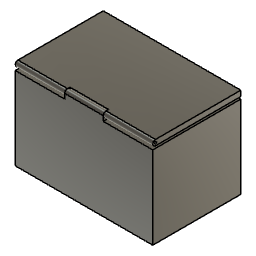
Speaker Holder Prototype v7 (Autodesk Fusion 360 design; units mm, degrees)
Autodesk Fusion 360 part; units mm, degrees
note: some values were not read from the file. Set by a fixed rule: which sketch regions a step uses.
sketch "Sketch1" plane through (0, 0, 0) normal (0, 0, 1) x (1, 0, 0)
  line L0 (-100, 50) -> (400, 50)
  line L1 (400, 50) -> (400, -150)
  line L2 (400, -150) -> (-100, -150)
  line L3 (-100, -150) -> (-100, 50)
  dimension "d1" = 500
  dimension "d2" = 200
  constraint horizontal L0
  constraint vertical L1
  constraint horizontal L2
  constraint vertical L3
  measures "d1" distance of L0.start L0.end
  measures "d2" distance of L0.start L2.end
extrude "Extrude1" add sketch "Sketch1" along normal blind 100 makes body 1
sketch "Sketch2" plane through (0, 0, 100) normal (0, 0, 1) x (-1, 0, 0)
  line L0 (100, 150) -> (-400, 150)
  line L1 (-400, 150) -> (-400, -50)
  line L2 (-400, -50) -> (100, -50)
  line L3 (100, -50) -> (100, 150)
  line L4 (90, -40) -> (-390, -40)
  line L5 (-390, -40) -> (-390, 140)
  line L6 (-390, 140) -> (90, 140)
  line L7 (90, 140) -> (90, -40)
  constraint horizontal L4
  constraint vertical L5
  constraint horizontal L6
  constraint vertical L7
extrude "Extrude2" cut sketch "Sketch2" against normal blind 90 contours L4 L5 L6 L7 bodies 1
sketch "Sketch3" plane through (0, 0, 100) normal (0, 0, 1) x (-1, 0, 0)
  line L0 (-390, -40) -> (-390, 140)
  line L1 (-390, 140) -> (90, 140)
  line L2 (90, 140) -> (90, -40)
  line L3 (90, -40) -> (-390, -40)
  line L4 (100, 150) -> (-400, 150)
  line L5 (-400, 150) -> (-400, -50)
  line L6 (-400, -50) -> (100, -50)
  line L7 (100, -50) -> (100, 150)
  line L8 (-30, 140) -> (-70, 140)
  line L9 (-70, 140) -> (-70, 150)
  line L10 (-70, 150) -> (-30, 150)
  line L11 (-30, 150) -> (-30, 140)
  line L12 (-320, 150) -> (-280, 150)
  line L13 (-280, 150) -> (-280, 140)
  line L14 (-280, 140) -> (-320, 140)
  line L15 (-320, 140) -> (-320, 150)
  constraint horizontal L8
  constraint vertical L9
  constraint horizontal L10
  constraint vertical L11
  constraint coincident L4 L9.end
  constraint coincident L1 L8.start
  constraint horizontal L12
  constraint vertical L13
  constraint horizontal L14
  constraint vertical L15
  constraint coincident L1 L13.end
  constraint coincident L4 L12.start
extrude "Extrude3" add sketch "Sketch3" along normal blind 10 contours L1 L4 L12 L13 L14 L15 bodies 1
sketch "Sketch4" plane through (0, 0, 100) normal (0, 0, 1) x (-1, 0, 0)
  line L0 (-280, 150) -> (-280, 140)
  line L1 (-280, 140) -> (90, 140)
  line L2 (90, 140) -> (90, -40)
  line L3 (90, -40) -> (-390, -40)
  line L4 (-390, -40) -> (-390, 140)
  line L5 (-390, 140) -> (-320, 140)
  line L6 (-320, 140) -> (-320, 150)
  line L7 (-320, 150) -> (-400, 150)
  line L8 (-400, 150) -> (-400, -50)
  line L9 (-400, -50) -> (100, -50)
  line L10 (100, -50) -> (100, 150)
  line L11 (100, 150) -> (-280, 150)
  line L12 (-30, 140) -> (-70, 140)
  line L13 (-70, 140) -> (-70, 150)
  line L14 (-70, 150) -> (-30, 150)
  line L15 (-30, 150) -> (-30, 140)
  constraint horizontal L12
  constraint vertical L13
  constraint horizontal L14
  constraint vertical L15
  constraint coincident L11 L13.end
  constraint coincident L1 L12.start
extrude "Extrude4" add sketch "Sketch4" along normal blind 10 contours L1 L11 L12 L13 L14 L15 bodies 1
sketch "Sketch5" plane through (0, 0, 0) normal (0, 0, 1) x (1, 0, 0)
  line L0 (-100, 50) -> (400, 50)
  line L1 (400, 50) -> (400, -150)
  line L2 (400, -150) -> (-100, -150)
  line L3 (-100, -150) -> (-100, 50)
  line L4 (500, 0) -> (1000, 0)
  line L5 (1000, 0) -> (1000, -200)
  line L6 (1000, -200) -> (500, -200)
  line L7 (500, -200) -> (500, 0)
  dimension "d11" = 500
  dimension "d12" = 200
  constraint horizontal L0
  constraint vertical L1
  constraint horizontal L2
  constraint vertical L3
  constraint horizontal L4
  constraint vertical L5
  constraint horizontal L6
  constraint vertical L7
  measures "d11" distance of L4.start L4.end
  measures "d12" distance of L4.start L6.end
extrude "Extrude5" add sketch "Sketch5" along normal blind 10 separate body contours L4 L5 L6 L7 makes body 2
move_body "Move1" bodies 2 to x (1, 0, 0) y (0, 1, 0) z (0, 0, 1) at (-600, 0, 110)
move_body "Move2" bodies 2 to x (1, 0, 0) y (0, 1, 0) z (0, 0, 1) at (0, 50, 0)
sketch "Sketch6" plane through (0, 0, 120) normal (0, 0, 1) x (-1, 0, 0)
  line L0 (100, 150) -> (-400, 150)
  line L1 (-400, 150) -> (-400, -50)
  line L2 (-400, -50) -> (100, -50)
  line L3 (100, -50) -> (100, 150)
  line L4 (-30, 150) -> (-70, 150)
  line L5 (-70, 150) -> (-70, 130)
  line L6 (-70, 130) -> (-30, 130)
  line L7 (-30, 130) -> (-30, 150)
  constraint horizontal L4
  constraint vertical L5
  constraint horizontal L6
  constraint vertical L7
  constraint coincident L0 L4.start
extrude "Extrude6" cut sketch "Sketch6" against normal blind 10 contours L0 L4 L5 L6 L7 bodies 2
sketch "Sketch7" plane through (0, 0, 120) normal (0, 0, 1) x (-1, 0, 0)
  line L0 (-70, 130) -> (-70, 150)
  line L1 (-70, 150) -> (-400, 150)
  line L2 (-400, 150) -> (-400, -50)
  line L3 (-400, -50) -> (100, -50)
  line L4 (100, -50) -> (100, 150)
  line L5 (100, 150) -> (-30, 150)
  line L6 (-30, 150) -> (-30, 130)
  line L7 (-30, 130) -> (-70, 130)
  line L8 (-280, 150) -> (-320, 150)
  line L9 (-320, 150) -> (-320, 130)
  line L10 (-320, 130) -> (-280, 130)
  line L11 (-280, 130) -> (-280, 150)
  constraint horizontal L8
  constraint vertical L9
  constraint horizontal L10
  constraint vertical L11
  constraint coincident L1 L8.start
extrude "Extrude7" cut sketch "Sketch7" against normal blind 10 contours L1 L8 L9 L10 L11 bodies 2
sketch "Sketch8" plane through (0, 0, 120) normal (0, 0, 1) x (-1, 0, 0)
  line L0 (-280, 150) -> (-280, 130)
  line L1 (-280, 130) -> (-320, 130)
  line L2 (-320, 130) -> (-320, 150)
  line L3 (-320, 150) -> (-400, 150)
  line L4 (-400, 150) -> (-400, -50)
  line L5 (-400, -50) -> (100, -50)
  line L6 (100, -50) -> (100, 150)
  line L7 (100, 150) -> (-30, 150)
  line L8 (-30, 150) -> (-30, 130)
  line L9 (-30, 130) -> (-70, 130)
  line L10 (-70, 130) -> (-70, 150)
  line L11 (-70, 150) -> (-280, 150)
  line L12 (100, 150) -> (10, 150)
  line L13 (10, 150) -> (10, 130)
  line L14 (10, 130) -> (100, 130)
  line L15 (100, 130) -> (100, 150)
  constraint horizontal L12
  constraint vertical L13
  constraint horizontal L14
  constraint vertical L15
  constraint coincident L6.end L7.start
extrude "Extrude8" cut sketch "Sketch8" against normal blind 10 contours L6 L7 L12 L13 L14 L15 bodies 2
sketch "Sketch9" plane through (0, 0, 120) normal (0, 0, 1) x (-1, 0, 0)
  line L0 (100, 130) -> (10, 130)
  line L1 (10, 130) -> (10, 150)
  line L2 (10, 150) -> (-30, 150)
  line L3 (-30, 150) -> (-30, 130)
  line L4 (-30, 130) -> (-70, 130)
  line L5 (-70, 130) -> (-70, 150)
  line L6 (-70, 150) -> (-280, 150)
  line L7 (-280, 150) -> (-280, 130)
  line L8 (-280, 130) -> (-320, 130)
  line L9 (-320, 130) -> (-320, 150)
  line L10 (-320, 150) -> (-400, 150)
  line L11 (-400, 150) -> (-400, -50)
  line L12 (-400, -50) -> (100, -50)
  line L13 (100, -50) -> (100, 130)
  line L14 (-110, 130) -> (-240, 130)
  line L15 (-240, 130) -> (-240, 150)
  line L16 (-240, 150) -> (-110, 150)
  line L17 (-110, 150) -> (-110, 130)
  constraint horizontal L14
  constraint vertical L15
  constraint horizontal L16
  constraint vertical L17
  constraint coincident L6 L15.end
extrude "Extrude9" cut sketch "Sketch9" against normal blind 10 contours L6 L14 L15 L16 L17 bodies 2
sketch "Sketch10" plane through (0, 0, 120) normal (0, 0, 1) x (-1, 0, 0)
  line L0 (-110, 150) -> (-110, 130)
  line L1 (-110, 130) -> (-240, 130)
  line L2 (-240, 130) -> (-240, 150)
  line L3 (-240, 150) -> (-280, 150)
  line L4 (-280, 150) -> (-280, 130)
  line L5 (-280, 130) -> (-320, 130)
  line L6 (-320, 130) -> (-320, 150)
  line L7 (-320, 150) -> (-400, 150)
  line L8 (-400, 150) -> (-400, -50)
  line L9 (-400, -50) -> (100, -50)
  line L10 (100, -50) -> (100, 130)
  line L11 (100, 130) -> (10, 130)
  line L12 (10, 130) -> (10, 150)
  line L13 (10, 150) -> (-30, 150)
  line L14 (-30, 150) -> (-30, 130)
  line L15 (-30, 130) -> (-70, 130)
  line L16 (-70, 130) -> (-70, 150)
  line L17 (-70, 150) -> (-110, 150)
  line L18 (-360, 130) -> (-400, 130)
  line L19 (-400, 130) -> (-400, 150)
  line L20 (-400, 150) -> (-360, 150)
  line L21 (-360, 150) -> (-360, 130)
  constraint horizontal L18
  constraint vertical L19
  constraint horizontal L20
  constraint vertical L21
  constraint coincident L7.end L8.start
extrude "Extrude10" cut sketch "Sketch10" against normal blind 10 contours L7 L8 L18 L19 L20 L21 bodies 2
move_body "Move3" bodies 2 to x (1, 0, 0) y (0, 1, 0) z (0, 0, 1) at (0, 0, -10)
move_body "Move4" bodies 2 to x (1, 0, 0) y (0, 1, 0) z (0, 0, 1) at (0, 280, 0)
extrude "Extrude11" add 5 faces at (373.3333, 150, 106.6667) (306.6667, 150, 106.6667) (153.3333, 150, 103.3333) (56.6667, 150, 106.6667) (-40, 150, 106.6667) along direction (0, -1, 0) blind 10 on bodies 2 bodies 2
move_body "Move5" bodies 2 to x (1, 0, 0) y (0, 1, 0) z (0, 0, 1) at (0, -280, 0)
hole "Hole1" at (-10, -145, 105) direction (1, 0, 0) diameter 8 depth 10000 tip angle 180 bodies 1 2
move_body "Move6" bodies 2 to x (1, 0, 0) y (0, 1, 0) z (0, 0, 1) at (0, 0, 10)
sketch "Sketch11" plane through (0, 50, 0) normal (0, 1, 0) x (-1, 0, 0)
  line L0 (-400, 0) -> (100, 0)
  line L1 (100, 0) -> (100, 100)
  line L2 (100, 100) -> (-400, 100)
  line L3 (-400, 100) -> (-400, 0)
  line L4 (-380, 80) -> (80, 80)
  line L5 (80, 80) -> (80, 20)
  line L6 (80, 20) -> (-380, 20)
  line L7 (-380, 20) -> (-380, 80)
  constraint horizontal L4
  constraint vertical L5
  constraint horizontal L6
  constraint vertical L7
extrude "Extrude12" cut sketch "Sketch11" against normal blind 10 contours L4 L5 L6 L7 bodies 1
sketch "Sketch12" plane through (0, 0, 0) normal (0, 0, 1) x (1, 0, 0)
  line L0 (0, 250) -> (125, 250)
  line L1 (125, 250) -> (125, 170)
  line L2 (125, 170) -> (0, 170)
  line L3 (0, 170) -> (0, 250)
  constraint horizontal L0
  constraint vertical L1
  constraint horizontal L2
  constraint vertical L3
extrude "Extrude13" add sketch "Sketch12" along normal blind 75 separate body makes body 3
sketch "Sketch13" plane through (0, 0, 75) normal (0, 0, 1) x (-1, 0, 0)
  line L0 (0, -170) -> (-125, -170)
  line L1 (-125, -170) -> (-125, -250)
  line L2 (-125, -250) -> (0, -250)
  line L3 (0, -250) -> (0, -170)
  line L4 (-5, -245) -> (-120, -245)
  line L5 (-120, -245) -> (-120, -175)
  line L6 (-120, -175) -> (-5, -175)
  line L7 (-5, -175) -> (-5, -245)
  constraint horizontal L4
  constraint vertical L5
  constraint horizontal L6
  constraint vertical L7
extrude "Extrude14" cut sketch "Sketch13" against normal blind 70 contours L4 L5 L6 L7 bodies 3
sketch "Sketch14" plane through (0, 250, 0) normal (0, 1, 0) x (-1, 0, 0)
  line L0 (-125, 0) -> (0, 0)
  line L1 (0, 0) -> (0, 75)
  line L2 (0, 75) -> (-125, 75)
  line L3 (-125, 75) -> (-125, 0)
  line L4 (-115, 65) -> (-10, 65)
  line L5 (-10, 65) -> (-10, 10)
  line L6 (-10, 10) -> (-115, 10)
  line L7 (-115, 10) -> (-115, 65)
  constraint horizontal L4
  constraint vertical L5
  constraint horizontal L6
  constraint vertical L7
extrude "Extrude15" cut sketch "Sketch14" against normal blind 5 contours L4 L5 L6 L7 bodies 3
sketch "Sketch15" plane through (0, 0, 0) normal (1, 0, 0) x (0, 1, 0)
sketch "Sketch16" plane through (0, 0, 0) normal (0, 0, 1) x (1, 0, 0)
  line L0 (-54.6306, 165.2352) -> (-179.6306, 165.2352)
  line L1 (-179.6306, 165.2352) -> (-179.6306, 245.2352)
  line L2 (-179.6306, 245.2352) -> (-54.6306, 245.2352)
  line L3 (-54.6306, 245.2352) -> (-54.6306, 165.2352)
  dimension "d38" = 125
  dimension "d39" = 80
  constraint horizontal L0
  constraint vertical L1
  constraint horizontal L2
  constraint vertical L3
  measures "d38" distance of L0.start L0.end
  measures "d39" distance of L0.start L2.end
extrude "Extrude16" add sketch "Sketch16" along normal blind 5 separate body makes body 4
move_body "Move7" bodies 4 to x (1, 0, 0) y (0, 1, 0) z (0, 0, 1) at (179.7, 0, 75)
move_body "Move8" bodies 4 to x (1, 0, 0) y (0, 1, 0) z (0, 0, 1) at (0, 5, 5)
move_body "Move9" bodies 1 to x (1, 0, 0) y (0, 1, 0) z (0, 0, 1) at (1000, 0, 0)
move_body "Move10" bodies 2 to x (1, 0, 0) y (0, 1, 0) z (0, 0, 1) at (1000, 0, 0)
move_body "Move11" bodies 4 3 to x (1, 0, 0) y (0, 1, 0) z (0, 0, 1) at (25, 0, 0)
move_body "Move12" bodies 4 to x (1, 0, 0) y (0, 1, 0) z (0, 0, 1) at (-130, 0, 0)
sketch "Sketch17" plane through (0, 0, 75) normal (0, 0, 1) x (-1, 0, 0)
  line L0 (-145, -245) -> (-145, -175)
  line L1 (-145, -175) -> (-30, -175)
  line L2 (-30, -175) -> (-30, -245)
  line L3 (-30, -245) -> (-145, -245)
  line L4 (-25, -170) -> (-150, -170)
  line L5 (-150, -170) -> (-150, -250)
  line L6 (-150, -250) -> (-25, -250)
  line L7 (-25, -250) -> (-25, -170)
  line L8 (-70, -175) -> (-105, -175)
  line L9 (-105, -175) -> (-105, -170)
  line L10 (-105, -170) -> (-70, -170)
  line L11 (-70, -170) -> (-70, -175)
  constraint horizontal L8
  constraint vertical L9
  constraint horizontal L10
  constraint vertical L11
  constraint coincident L1 L8.start
extrude "Extrude17" add sketch "Sketch17" along normal blind 5 contours L1 L4 L8 L9 L10 L11 bodies 3
move_body "Move13" bodies 4 to x (1, 0, 0) y (0, 1, 0) z (0, 0, 1) at (130, 0, 0)
sketch "Sketch18" plane through (0, 0, 85) normal (0, 0, 1) x (-1, 0, 0)
  line L0 (-150.0694, -250.2352) -> (-25.0694, -250.2352)
  line L1 (-25.0694, -250.2352) -> (-25.0694, -170.2352)
  line L2 (-25.0694, -170.2352) -> (-150.0694, -170.2352)
  line L3 (-150.0694, -170.2352) -> (-150.0694, -250.2352)
  line L4 (-70, -175) -> (-105.1562, -175)
  line L5 (-105.1562, -175) -> (-105.1562, -170.2352)
  line L6 (-105.1562, -170.2352) -> (-70, -170.2352)
  line L7 (-70, -170.2352) -> (-70, -175)
  constraint horizontal L4
  constraint vertical L5
  constraint horizontal L6
  constraint vertical L7
  constraint coincident L2 L5.end
extrude "Extrude18" cut sketch "Sketch18" against normal blind 5 contours L2 L4 L5 L6 L7 bodies 4
move_body "Move14" bodies 4 to x (1, 0, 0) y (0, 1, 0) z (0, 0, 1) at (0, 0, -5)
move_body "Move15" bodies 4 to x (1, 0, 0) y (0, 1, 0) z (0, 0, 1) at (0, -0.2352, 0)
move_body "Move16" bodies 4 to x (1, 0, 0) y (0, 1, 0) z (0, 0, 1) at (-0.0694, 0, 0)
sketch "Sketch19" plane through (25, 0, 0) normal (-1, 0, 0) x (0, -1, 0)
  line L0 (-250, 75) -> (-170, 75)
  line L1 (-170, 75) -> (-170, 80)
  line L2 (-170, 80) -> (-250, 80)
  line L3 (-250, 80) -> (-250, 75)
  line L4 (-170, 77.5) -> (-172.5, 77.5)
  dimension "d46" = 2.5
  constraint midpoint L1 L4.start
  constraint perpendicular L1 L4
  measures "d46" distance of L4.start L4.end
hole "Hole2" at (25, 172.5, 77.5) direction (1, 0, 0) diameter 2.2 depth 1000000 tip angle 180 bodies 3 4
sketch "Sketch20" plane through (25, 0, 0) normal (-1, 0, 0) x (0, -1, 0)
  circle A0 centre (-172.5, 77.5) radius 1.1
  line L0 (-250, 75) -> (-170, 75)
  line L1 (-170, 75) -> (-170, 80)
  line L2 (-170, 80) -> (-250, 80)
  line L3 (-250, 80) -> (-250, 75)
sketch "Sketch21" plane through (25, 0, 0) normal (-1, 0, 0) x (0, -1, 0)
move_body "Move17" bodies 4 to x (1, 0, 0) y (0, 1, 0) z (0, 0, 1) at (0, 0, 5)
sketch "Sketch22" plane through (150, 0, 0) normal (1, 0, 0) x (0, 1, 0)
  circle A0 centre (172.5, 82.5) radius 1.1
  line L0 (170, 80) -> (250, 80)
  line L1 (250, 80) -> (250, 85)
  line L2 (250, 85) -> (170, 85)
  line L3 (170, 85) -> (170, 80)
  line L4 (175, 80) -> (172.4857, 80)
  line L5 (172.4857, 80) -> (172.4857, 85)
  line L6 (172.4857, 85) -> (175, 85)
  line L7 (175, 85) -> (175, 80)
  circle A1 centre (172.5, 82.5) radius 2.5
  constraint horizontal L4
  constraint vertical L5
  constraint horizontal L6
  constraint vertical L7
  constraint coincident L2 L5.end
  constraint concentric A0 A1
  constraint tangent L3 A1
extrude "Extrude19" cut sketch "Sketch22" against normal blind 200 contours L2 L3 A1 | L0 L3 A1 bodies 4
sketch "Sketch23" plane through (105, 0, 0) normal (1, 0, 0) x (0, 1, 0)
  circle A0 centre (172.5, 77.5) radius 1.1
  line L0 (170, 75) -> (175, 75)
  line L1 (175, 75) -> (175, 80)
  line L2 (175, 80) -> (170, 80)
  line L3 (170, 80) -> (170, 75)
  line L4 (170, 77.5) -> (175, 77.5)
  line L5 (175, 77.5) -> (175, 75)
  line L6 (175, 75) -> (170, 75)
  line L7 (170, 75) -> (170, 77.5)
  circle A1 centre (172.5, 77.5) radius 2.5
  constraint horizontal L4
  constraint vertical L5
  constraint horizontal L6
  constraint vertical L7
  constraint coincident L0.end L1.start
  constraint midpoint L3 L4.start
  constraint concentric A0 A1
  constraint coincident L4.start A1
extrude "Extrude20" cut sketch "Sketch23" against normal blind 200 contours L1 L2 A1 | L2 L3 A1 bodies 3
move_body "Move18" bodies 4 to x (1, 0, 0) y (0, 1, 0) z (0, 0, 1) at (0, 0, 5)
extrude "Extrude21" cut 1 faces at (68.3333, 248.3333, 75) along direction (0, 0, -1) blind 2 on bodies 3 bodies 3
extrude "Extrude22" add 1 faces at (66.6667, 223.3333, 0) along direction (0, 0, -1) blind 2 on bodies 3 bodies 3
move_body "Move19" bodies 4 to x (1, 0, 0) y (0, 1, 0) z (0, 0, 1) at (0, 0, -10)
hidden bodies 1 2
equation "d47 = 1.000E+06 mm"
